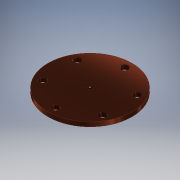
# Autodesk Inventor part: 1mm Electrode
Saved by Autodesk Inventor 2017.3 (Build 213256000, 256)
## iProperties
Created: 2017-02-02
Part Number: 1mm Electrode
Material: Generic
Document SubType Name: Modeling
Designer: Mac
Density: 1 g/cm^3
Appearance: Copper - Polished
Author: Mac
Autodesk Inventor part; units mm, degrees
ref_plane "YZ Plane" through (0, 0, 0) normal (1, 0, 0) x (0, 1, 0)
ref_plane "XZ Plane" through (0, 0, 0) normal (0, 1, 0) x (-1, 0, 0)
ref_plane "XY Plane" through (0, 0, 0) normal (0, 0, 1) x (1, 0, 0)
sketch "Sketch1" plane through (0, 0, 0) normal (1, 0, 0) x (0, 1, 0)
  circle A0 centre (0, 0) radius 9.5
  dimension "d0" = 19
  constraints: 1 centre point, 1 coincident
  measures "d0" diameter of A0
extrude "Extrusion1" add sketch "Sketch1" along normal blind 1
sketch "Sketch2" plane through (1, 0, 0) normal (1, 0, 0) x (0, 0, -1)
  circle A0 centre (0, 0) radius 0.5
  circle A1 centre (0, 7.81) radius 0.835
  circle A2 centre (0, -7.81) radius 0.835
  circle A3 centre (6.7637, 3.905) radius 0.835
  circle A4 centre (6.7637, -3.905) radius 0.835
  circle A5 centre (-6.7637, -3.905) radius 0.835
  circle A6 centre (-6.7637, 3.905) radius 0.835
  dimension "d3" = 1
  dimension "d4" = 1.67
  dimension "d5" = 1.67
  dimension "d6" = 1.67
  dimension "d7" = 1.67
  dimension "d8" = 1.67
  dimension "d9" = 1.67
  constraints: 7 centre point, 1 coincident
  measures "d3" diameter of A0
  measures "d4" diameter of A1
  measures "d5" diameter of A2
  measures "d6" diameter of A3
  measures "d7" diameter of A4
  measures "d8" diameter of A5
  measures "d9" diameter of A6
extrude "Extrusion2" cut sketch "Sketch2" against normal blind 1
move or copy body "Move Body1" bodies to move or copy 1 copy no rotation origin (0, 0, 0) rotation axis (0, 1, 0) rotation angle 90
sketch "Sketch3" plane through (0, 0, 0) normal (0, 0, 1) x (1, 0, 0)
  point P0 (0, 0)
body "Solid1"
